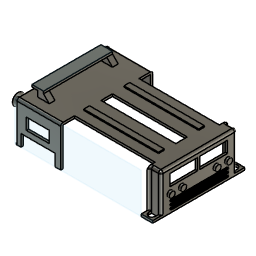
coverrrrr v1 v2 (Autodesk Fusion 360 design; units mm, degrees)
Autodesk Fusion 360 part; units mm, degrees
note: some values were not read from the file. Set by a fixed rule: which sketch regions a step uses.
sketch "Sketch1" plane through (0, 0, 0) normal (0, 0, 1) x (1, 0, 0)
  line L0 (0, 0) -> (120, 0)
  line L1 (120, 0) -> (120, 80)
  line L2 (120, 80) -> (0, 80)
  line L3 (0, 80) -> (0, 0)
  dimension "d1" = 120
  dimension "d2" = 80
  constraint horizontal L0
  constraint vertical L1
  constraint horizontal L2
  constraint vertical L3
  constraint coincident L0.start L3.end
  measures "d1" distance of L0.start L0.end
  measures "d2" distance of L0.start L2.end
extrude "Extrude1" add sketch "Sketch1" along normal blind 35
sketch "Sketch2" plane through (0, 0, 35) normal (0, 0, 1) x (-1, 0, 0)
  line L0 (0, -80) -> (0, 0)
  line L1 (0, 0) -> (-120, 0)
  line L2 (-120, 0) -> (-120, -80)
  line L3 (-120, -80) -> (0, -80)
  line L4 (-120, 0) -> (-110, 0)
  line L5 (-110, 0) -> (-110, -7)
  line L6 (-110, -7) -> (-120, -7)
  line L7 (-120, -7) -> (-120, 0)
  dimension "d5" = 10
  dimension "d6" = 7
  constraint horizontal L4
  constraint vertical L5
  constraint horizontal L6
  constraint vertical L7
  constraint coincident L1.end L2.start
  measures "d5" distance of L1.end L4.end
  measures "d6" distance of L1.end L6.end
extrude "Extrude2" cut sketch "Sketch2" against normal blind 33 contours L1 L2 L4 L5 L6 L7
sketch "Sketch3" plane through (0, 0, 35) normal (0, 0, 1) x (-1, 0, 0)
  line L0 (-110, 0) -> (-110, -7)
  line L1 (-110, -7) -> (-120, -7)
  line L2 (-120, -7) -> (-120, -80)
  line L3 (-120, -80) -> (0, -80)
  line L4 (0, -80) -> (0, 0)
  line L5 (0, 0) -> (-110, 0)
  line L6 (-120, -80) -> (-110, -80)
  line L7 (-110, -80) -> (-110, -73)
  line L8 (-110, -73) -> (-120, -73)
  line L9 (-120, -73) -> (-120, -80)
  dimension "d9" = 10
  dimension "d10" = 7
  constraint horizontal L6
  constraint vertical L7
  constraint horizontal L8
  constraint vertical L9
  constraint coincident L2.end L3.start
  measures "d9" distance of L2.end L6.end
  measures "d10" distance of L2.end L8.end
extrude "Extrude3" cut sketch "Sketch3" against normal blind 33 contours L2 L3 L6 L7 L8 L9
sketch "Sketch4" plane through (0, 0, 2) normal (0, 0, 1) x (-1, 0, 0)
  line L0 (-120, -7) -> (-110, -7)
  line L1 (-110, -7) -> (-110, 0)
  line L2 (-110, 0) -> (-120, 0)
  line L3 (-120, 0) -> (-120, -7)
  line L4 (-110, -2) -> (-113, -2)
  line L5 (-113, -2) -> (-113, 0)
  circle A0 centre (-115, -4) radius 2.75
  dimension "d13" = 5.5
  constraint coincident L1 L4.start
  constraint perpendicular L1 L4
  constraint coincident L2 L5.end
  constraint perpendicular L2 L5
  measures "d13" diameter of A0
extrude "Extrude4" cut sketch "Sketch4" against normal blind 5 contours A0
sketch "Sketch5" plane through (0, 0, 2) normal (0, 0, 1) x (-1, 0, 0)
  line L0 (-120, -73) -> (-120, -80)
  line L1 (-120, -80) -> (-110, -80)
  line L2 (-110, -80) -> (-110, -73)
  line L3 (-110, -73) -> (-120, -73)
  line L4 (-110, -78) -> (-113, -78)
  line L5 (-113, -78) -> (-113, -80)
  circle A0 centre (-115, -76) radius 2.75
  dimension "d16" = 5.5
  constraint coincident L2 L4.start
  constraint perpendicular L2 L4
  constraint coincident L1 L5.end
  constraint perpendicular L1 L5
  measures "d16" diameter of A0
extrude "Extrude5" cut sketch "Sketch5" against normal blind 4 contours A0
sketch "Sketch6" plane through (0, 0, 0) normal (0, -1, 0) x (1, 0, 0)
  line L0 (110, 2) -> (110, 35)
  line L1 (110, 35) -> (0, 35)
  line L2 (0, 35) -> (0, 0)
  line L3 (0, 0) -> (120, 0)
  line L4 (120, 0) -> (120, 2)
  line L5 (120, 2) -> (110, 2)
shell "Shell1" thickness 2 removed faces 1 at (37.5759, 28.5164, 0)
sketch "Sketch7" plane through (0, 0, 0) normal (0, -1, 0) x (1, 0, 0)
sketch "Sketch8" plane through (0, 0, 0) normal (0, -1, 0) x (1, 0, 0)
  line L0 (0, 0) -> (40, 0)
  line L1 (40, 0) -> (105, 0)
  line L2 (105, 0) -> (105, 25)
  line L3 (105, 25) -> (40, 25)
  line L4 (40, 25) -> (40, 0)
  dimension "d20" = 40
  dimension "d21" = 65
  dimension "d22" = 25
  constraint coincident L0.start origin
  constraint horizontal L0
  constraint horizontal L1
  constraint vertical L2
  constraint horizontal L3
  constraint vertical L4
  measures "d20" distance of L0.start L0.end
  measures "d21" distance of L0.end L1.end
  measures "d22" distance of L0.end L3.end
extrude "Extrude6" cut sketch "Sketch8" against normal blind 150
sketch "Sketch9" plane through (0, 0, 0) normal (-1, 0, 0) x (0, -1, 0)
  line L0 (-80, 0) -> (0, 0)
  line L1 (0, 0) -> (0, 35)
  line L2 (0, 35) -> (-80, 35)
  line L3 (-80, 35) -> (-80, 0)
  line L4 (-5, 0) -> (-75, 0)
  line L5 (-75, 0) -> (-75, 30)
  line L6 (-75, 30) -> (-5, 30)
  line L7 (-5, 30) -> (-5, 0)
  constraint horizontal L4
  constraint vertical L5
  constraint horizontal L6
  constraint vertical L7
  constraint coincident L0 L4.start
extrude "Extrude7" cut sketch "Sketch9" against normal blind 15 contours L0 L4 L5 L6 L7
fillet "Fillet1" radius 10 6 edges at (105, 1, 25) (40, 1, 25) (40, 79, 25) (105, 79, 25) (1, 5, 30) (1, 75, 30)
fillet "Fillet2" radius 2 16 edges at (55, 80, 35) (0, 80, 17.5) (0, 40, 35) (0, 0, 17.5) (55, 0, 35) (110, 3.5, 35) (115, 7, 35) (120, 40, 35) (115, 73, 35) (110, 76.5, 35) (120, 73, 18.5) (110, 80, 18.5) (110, 73, 18.5) (110, 0, 18.5) (110, 7, 18.5) (120, 7, 18.5)
sketch "Sketch10" plane through (0, 0, 35) normal (0, 0, 1) x (-1, 0, 0)
  arc A0 (-108, -75) -> (-112, -71) centre (-112, -75) ccw
  line L0 (-108, -75) -> (-108, -78)
  line L1 (-108, -78) -> (-2, -78)
  line L2 (-2, -78) -> (-2, -2)
  line L3 (-2, -2) -> (-108, -2)
  line L4 (-108, -2) -> (-108, -5)
  arc A1 (-112, -9) -> (-108, -5) centre (-112, -5) ccw
  line L5 (-112, -9) -> (-118, -9)
  line L6 (-118, -9) -> (-118, -71)
  line L7 (-118, -71) -> (-112, -71)
  line L8 (-20, -10) -> (-10, -10)
  line L9 (-10, -10) -> (-10, -15)
  line L10 (-10, -15) -> (-20, -15)
  line L11 (-20, -15) -> (-20, -10)
  line L12 (-20, -65) -> (-10, -65)
  line L13 (-10, -65) -> (-10, -70)
  line L14 (-10, -70) -> (-20, -70)
  line L15 (-20, -70) -> (-20, -65)
  constraint horizontal L8
  constraint vertical L9
  constraint horizontal L10
  constraint vertical L11
  constraint horizontal L12
  constraint vertical L13
  constraint horizontal L14
  constraint vertical L15
extrude "Extrude8" add sketch "Sketch10" along normal blind 5 contours L8 L9 L10 L11 | L12 L13 L14 L15
sketch "Sketch11" plane through (0, 0, 40) normal (0, 0, 1) x (-1, 0, 0)
  line L0 (-20, -15) -> (-10, -15)
  line L1 (-10, -15) -> (-10, -10)
  line L2 (-10, -10) -> (-20, -10)
  line L3 (-20, -10) -> (-20, -15)
  line L4 (-15, -10) -> (-5, -10)
  line L5 (-5, -10) -> (-5, -70)
  line L6 (-5, -70) -> (-15, -70)
  line L7 (-15, -70) -> (-15, -10)
  constraint horizontal L4
  constraint vertical L5
  constraint horizontal L6
  constraint vertical L7
  constraint midpoint L2 L4.start
extrude "Extrude9" add sketch "Sketch11" along normal blind 2 contours L0 L1 L2 L4 L7 | L0 L1 L4 L5 L6 L7
sketch "Sketch12" plane through (0, 0, 0) normal (0, -1, 0) x (1, 0, 0)
  line L0 (40, 30) -> (100, 30)
  line L1 (100, 30) -> (100, 28)
  line L2 (100, 28) -> (40, 28)
  line L3 (40, 28) -> (40, 30)
  constraint horizontal L0
  constraint vertical L1
  constraint horizontal L2
  constraint vertical L3
sketch "Sketch13" plane through (0, 80, 0) normal (0, 1, 0) x (-1, 0, 0)
  line L0 (-2, 0) -> (-2, 33)
  line L1 (-2, 33) -> (-108, 33)
  line L2 (-108, 33) -> (-108, 2)
  line L3 (-108, 2) -> (-120, 2)
  line L4 (-120, 2) -> (-120, 0)
  line L5 (-120, 0) -> (-105, 0)
  line L6 (-105, 0) -> (-105, 15)
  arc A0 (-95, 25) -> (-105, 15) centre (-95, 15) ccw
  line L7 (-95, 25) -> (-50, 25)
  arc A1 (-40, 15) -> (-50, 25) centre (-50, 15) ccw
  line L8 (-40, 15) -> (-40, 0)
  line L9 (-40, 0) -> (-2, 0)
  line L10 (-40, 30) -> (-100, 30)
  line L11 (-100, 30) -> (-100, 28)
  line L12 (-100, 28) -> (-40, 28)
  line L13 (-40, 28) -> (-40, 30)
  constraint horizontal L10
  constraint vertical L11
  constraint horizontal L12
  constraint vertical L13
extrude "Extrude10" add sketch "Sketch12" along normal blind 20
extrude "Extrude11" add sketch "Sketch13" along normal blind 20 contours L10 L11 L12 L13
sketch "Sketch14" plane through (0, 0, 30) normal (0, 0, 1) x (-1, 0, 0)
  line L0 (-40, -80) -> (-100, -80)
  line L1 (-100, -80) -> (-100, -100)
  line L2 (-100, -100) -> (-40, -100)
  line L3 (-40, -100) -> (-40, -80)
  line L4 (-100, 0) -> (-40, 20)
  line L5 (-40, 20) -> (-100, 20)
  line L6 (-100, 20) -> (-100, 0)
  line L7 (-100, -80) -> (-40, -100)
  line L8 (-100, -100) -> (-100, -80)
  constraint horizontal L5
  constraint perpendicular L5 L6
  constraint coincident L0.end L1.start
  constraint coincident L2.end L3.start
  constraint coincident L1.end L2.start
extrude "Extrude12" cut sketch "Sketch14" against normal blind 10 contours L1 L2 L7 L8 | L4 L5 L6
sketch "Sketch15" plane through (0, 0, 30) normal (0, 0, 1) x (-1, 0, 0)
  line L0 (-100, -80) -> (-40, -100)
  line L1 (-40, -100) -> (-40, -80)
  line L2 (-40, -80) -> (-100, -80)
  circle A0 centre (-40, -90) radius 10
  circle A1 centre (-40, 10) radius 10
  constraint midpoint L1 A0.centre
  constraint coincident L1.end A0
extrude "Extrude13" cut sketch "Sketch15" against normal blind 10 contours L0 L1 A0 | L1 A0 | A1
sketch "Sketch16" plane through (0, 0, 0) normal (-1, 0, 0) x (0, -1, 0)
  line L0 (-78, 33) -> (-78, 0)
  line L1 (-78, 0) -> (-75, 0)
  line L2 (-75, 0) -> (-75, 20)
  arc A0 (-65, 30) -> (-75, 20) centre (-65, 20) ccw
  line L3 (-65, 30) -> (-15, 30)
  arc A1 (-5, 20) -> (-15, 30) centre (-15, 20) ccw
  line L4 (-5, 20) -> (-5, 0)
  line L5 (-5, 0) -> (-2, 0)
  line L6 (-2, 0) -> (-2, 33)
  line L7 (-2, 33) -> (-78, 33)
  circle A2 centre (-72.0711, 27.0711) radius 5
  circle A3 centre (-7.9289, 27.0711) radius 5
  dimension "d43" = 10
  dimension "d44" = 10
  constraint midpoint A0 A2.centre
  constraint midpoint A1 A3.centre
  measures "d43" diameter of A2
  measures "d44" diameter of A3
extrude "Extrude14" add sketch "Sketch16" along normal blind 5 contours A0 A2 | A0 A2 | A1 A3 | A1 A3
sketch "Sketch17" plane through (120, 0, 0) normal (1, 0, 0) x (0, 1, 0)
  line L0 (80, 2) -> (71, 2)
  line L1 (71, 2) -> (71, 33)
  line L2 (71, 33) -> (9, 33)
  line L3 (9, 33) -> (9, 2)
  line L4 (9, 2) -> (0, 2)
  line L5 (0, 2) -> (0, 0)
  line L6 (0, 0) -> (80, 0)
  line L7 (80, 0) -> (80, 2)
  line L8 (15, 30) -> (65, 30)
  line L9 (65, 30) -> (65, 20)
  line L10 (65, 20) -> (15, 20)
  line L11 (15, 20) -> (15, 30)
  constraint horizontal L8
  constraint vertical L9
  constraint horizontal L10
  constraint vertical L11
extrude "Extrude15" cut sketch "Sketch17" against normal blind 10 contours L8 L9 L10 L11
sketch "Sketch18" plane through (120, 0, 0) normal (1, 0, 0) x (0, 1, 0)
  line L0 (65, 30) -> (65, 20)
  line L1 (65, 20) -> (15, 20)
  line L2 (15, 20) -> (15, 30)
  line L3 (15, 30) -> (65, 30)
  line L4 (80, 2) -> (71, 2)
  line L5 (71, 2) -> (71, 33)
  line L6 (71, 33) -> (9, 33)
  line L7 (9, 33) -> (9, 2)
  line L8 (9, 2) -> (0, 2)
  line L9 (0, 2) -> (0, 0)
  line L10 (0, 0) -> (80, 0)
  line L11 (80, 0) -> (80, 2)
  circle A0 centre (15, 15) radius 2.5
  circle A1 centre (25, 15) radius 2.5
  circle A2 centre (65, 15) radius 2.5
  circle A3 centre (55, 15) radius 2.5
  dimension "d49" = 5
  dimension "d50" = 5
  dimension "d51" = 5
  dimension "d52" = 5
  measures "d49" diameter of A0
  measures "d50" diameter of A1
  measures "d51" diameter of A2
  measures "d52" diameter of A3
extrude "Extrude16" add sketch "Sketch18" along normal blind 2 contours A0 | A1 | A2 | A3
sketch "Sketch19" plane through (120, 0, 0) normal (1, 0, 0) x (0, 1, 0)
  circle A0 centre (65, 15) radius 2.5
  circle A1 centre (15, 15) radius 2.5
  circle A2 centre (55, 15) radius 2.5
  circle A3 centre (25, 15) radius 2.5
  line L0 (65, 30) -> (65, 20)
  line L1 (65, 20) -> (15, 20)
  line L2 (15, 20) -> (15, 30)
  line L3 (15, 30) -> (65, 30)
  line L4 (80, 2) -> (71, 2)
  line L5 (71, 2) -> (71, 33)
  line L6 (71, 33) -> (9, 33)
  line L7 (9, 33) -> (9, 2)
  line L8 (9, 2) -> (0, 2)
  line L9 (0, 2) -> (0, 0)
  line L10 (0, 0) -> (80, 0)
  line L11 (80, 0) -> (80, 2)
sketch "Sketch20" plane through (120, 0, 0) normal (1, 0, 0) x (0, 1, 0)
  line L0 (15, 10) -> (65, 10)
  line L1 (65, 10) -> (65, 9)
  line L2 (65, 9) -> (15, 9)
  line L3 (15, 9) -> (15, 10)
  line L4 (65, 7) -> (15, 7)
  line L5 (15, 7) -> (15, 6)
  line L6 (15, 6) -> (65, 6)
  line L7 (65, 6) -> (65, 7)
  line L8 (15, 4) -> (65, 4)
  line L9 (65, 4) -> (65, 3)
  line L10 (65, 3) -> (15, 3)
  line L11 (15, 3) -> (15, 4)
  constraint horizontal L0
  constraint vertical L1
  constraint horizontal L2
  constraint vertical L3
  constraint horizontal L4
  constraint vertical L5
  constraint horizontal L6
  constraint vertical L7
  constraint horizontal L8
  constraint vertical L9
  constraint horizontal L10
  constraint vertical L11
extrude "Extrude17" add sketch "Sketch20" along normal blind 1
sketch "Sketch21" plane through (0, 0, 20) normal (0, 0, 1) x (-1, 0, 0)
  line L0 (-118, -65) -> (-118, -15)
  line L1 (-118, -15) -> (-120, -15)
  line L2 (-120, -15) -> (-120, -65)
  line L3 (-120, -65) -> (-118, -65)
  line L4 (-118, -27) -> (-118, -53)
  line L5 (-120, -27) -> (-120, -40)
  line L6 (-118, -39) -> (-120, -39)
  line L7 (-120, -39) -> (-120, -41)
  line L8 (-120, -41) -> (-118, -41)
  line L9 (-118, -41) -> (-118, -39)
  constraint coincident L0 L4.start
  constraint coincident L0 L4.end
  constraint coincident L2 L5.start
  constraint midpoint L2 L5.end
  constraint horizontal L6
  constraint vertical L7
  constraint horizontal L8
  constraint vertical L9
  constraint coincident L2 L7.end
  constraint coincident L4 L6.start
extrude "Extrude18" add sketch "Sketch21" along normal blind 10 contours L0 L2 L4 L5 L6 L7 L8 L9
sketch "Sketch22" plane through (0, 0, 35) normal (0, 0, 1) x (-1, 0, 0)
  line L0 (-20, -15) -> (-20, -10)
  line L1 (-20, -10) -> (-10, -10)
  line L2 (-10, -10) -> (-10, -15)
  line L3 (-10, -15) -> (-20, -15)
  line L4 (-20, -70) -> (-20, -65)
  line L5 (-20, -65) -> (-10, -65)
  line L6 (-10, -65) -> (-10, -70)
  line L7 (-10, -70) -> (-20, -70)
  arc A0 (-108, -75) -> (-112, -71) centre (-112, -75) ccw
  line L8 (-108, -75) -> (-108, -78)
  line L9 (-108, -78) -> (-2, -78)
  line L10 (-2, -78) -> (-2, -2)
  line L11 (-2, -2) -> (-108, -2)
  line L12 (-108, -2) -> (-108, -5)
  arc A1 (-112, -9) -> (-108, -5) centre (-112, -5) ccw
  line L13 (-112, -9) -> (-118, -9)
  line L14 (-118, -9) -> (-118, -71)
  line L15 (-118, -71) -> (-112, -71)
  line L16 (-40, -60) -> (-105, -60)
  line L17 (-105, -60) -> (-105, -55)
  line L18 (-105, -55) -> (-40, -55)
  line L19 (-40, -55) -> (-40, -60)
  line L20 (-40, -20) -> (-105, -20)
  line L21 (-105, -20) -> (-105, -25)
  line L22 (-105, -25) -> (-40, -25)
  line L23 (-40, -25) -> (-40, -20)
  constraint horizontal L16
  constraint vertical L17
  constraint horizontal L18
  constraint vertical L19
  constraint horizontal L20
  constraint vertical L21
  constraint horizontal L22
  constraint vertical L23
extrude "Extrude19" add sketch "Sketch22" along normal blind 1 contours L16 L17 L18 L19 | L20 L21 L22 L23
sketch "Sketch23" plane through (-5, 0, 0) normal (-1, 0, 0) x (0, -1, 0)
  circle A0 centre (-7.9289, 27.0711) radius 5
  circle A1 centre (-7.9289, 27.0711) radius 4
  dimension "d61" = 8
  constraint concentric A0 A1
  measures "d61" diameter of A1
extrude "Extrude20" cut sketch "Sketch23" against normal blind 4 contours A1
sketch "Sketch24" plane through (-5, 0, 0) normal (-1, 0, 0) x (0, -1, 0)
  circle A0 centre (-72.0711, 27.0711) radius 5
  circle A1 centre (-72.0711, 27.0711) radius 4
  dimension "d64" = 8
  constraint concentric A0 A1
  measures "d64" diameter of A1
extrude "Extrude21" cut sketch "Sketch24" against normal blind 4 contours A1
sketch "Sketch25" plane through (0, 10, 0) normal (0, -1, 0) x (1, 0, 0)
  line L0 (10, 35) -> (20, 35)
  line L1 (20, 35) -> (20, 40)
  line L2 (20, 40) -> (15, 40)
  line L3 (15, 40) -> (15, 42)
  line L4 (15, 42) -> (5, 42)
  line L5 (5, 42) -> (5, 40)
  line L6 (5, 40) -> (10, 40)
  line L7 (10, 40) -> (10, 35)
  line L8 (15, 40) -> (20, 35)
  line L9 (20, 40) -> (15, 40)
  constraint coincident L2.end L3.start
  constraint coincident L0.end L1.start
  constraint coincident L1.end L2.start
extrude "Extrude22" cut sketch "Sketch25" against normal blind 63 contours L1 L2 L8 L9
sketch "Sketch26" plane through (0, 0, 42) normal (0, 0, 1) x (-1, 0, 0)
  line L0 (-15, -70) -> (-5, -70)
  line L1 (-5, -70) -> (-5, -10)
  line L2 (-5, -10) -> (-15, -10)
  line L3 (-15, -10) -> (-15, -70)
extrude "Extrude23" cut 2 faces at (66.5474, -5.5104, 30) (66.5474, 85.5104, 30) along direction (0, 0, -1) blind 10
sketch "Sketch27" plane through (0, 80, 0) normal (0, 1, 0) x (-1, 0, 0)
  arc A0 (-40, 15) -> (-50, 25) centre (-50, 15) ccw
  line L0 (-40, 15) -> (-40, 0)
  line L1 (-40, 0) -> (-2, 0)
  line L2 (-2, 0) -> (-2, 33)
  line L3 (-2, 33) -> (-108, 33)
  line L4 (-108, 33) -> (-108, 2)
  line L5 (-108, 2) -> (-120, 2)
  line L6 (-120, 2) -> (-120, 0)
  line L7 (-120, 0) -> (-105, 0)
  line L8 (-105, 0) -> (-105, 15)
  arc A1 (-95, 25) -> (-105, 15) centre (-95, 15) ccw
  line L9 (-95, 25) -> (-50, 25)
  line L10 (-30, 25) -> (-10, 25)
  line L11 (-10, 25) -> (-10, 15)
  line L12 (-10, 15) -> (-30, 15)
  line L13 (-30, 15) -> (-30, 25)
  constraint horizontal L10
  constraint vertical L11
  constraint horizontal L12
  constraint vertical L13
extrude "Extrude24" cut sketch "Sketch27" against normal blind 90 contours L10 L11 L12 L13
sketch "Sketch28" plane through (0, 0, 35) normal (0, 0, 1) x (-1, 0, 0)
  line L0 (-20, -65) -> (-10, -65)
  line L1 (-10, -65) -> (-10, -70)
  line L2 (-10, -70) -> (-20, -70)
  line L3 (-20, -70) -> (-20, -65)
  line L4 (-40, -55) -> (-40, -60)
  line L5 (-40, -60) -> (-105, -60)
  line L6 (-105, -60) -> (-105, -55)
  line L7 (-105, -55) -> (-40, -55)
  line L8 (-40, -25) -> (-105, -25)
  line L9 (-105, -25) -> (-105, -20)
  line L10 (-105, -20) -> (-40, -20)
  line L11 (-40, -20) -> (-40, -25)
  line L12 (-20, -15) -> (-20, -10)
  line L13 (-20, -10) -> (-10, -10)
  line L14 (-10, -10) -> (-10, -15)
  line L15 (-10, -15) -> (-20, -15)
  arc A0 (-108, -75) -> (-112, -71) centre (-112, -75) ccw
  line L16 (-108, -75) -> (-108, -78)
  line L17 (-108, -78) -> (-2, -78)
  line L18 (-2, -78) -> (-2, -2)
  line L19 (-2, -2) -> (-108, -2)
  line L20 (-108, -2) -> (-108, -5)
  arc A1 (-112, -9) -> (-108, -5) centre (-112, -5) ccw
  line L21 (-112, -9) -> (-118, -9)
  line L22 (-118, -9) -> (-118, -71)
  line L23 (-118, -71) -> (-112, -71)
  line L24 (-40, -45) -> (-105, -45)
  line L25 (-105, -45) -> (-105, -35)
  line L26 (-105, -35) -> (-40, -35)
  line L27 (-40, -35) -> (-40, -45)
  constraint horizontal L24
  constraint vertical L25
  constraint horizontal L26
  constraint vertical L27
extrude "Extrude25" cut sketch "Sketch28" against normal blind 5 contours L24 L25 L26 L27
sketch "Sketch29" plane through (0, 0, 0) normal (0, -1, 0) x (1, 0, 0)
  line L0 (40, 0) -> (110, 0)
  line L1 (110, 0) -> (110, 40)
  line L2 (110, 40) -> (40, 40)
  line L3 (40, 40) -> (40, 0)
  constraint horizontal L0
  constraint vertical L1
  constraint horizontal L2
  constraint vertical L3
extrude "Extrude26" cut sketch "Sketch29" against normal blind 12
sketch "Sketch30" plane through (0, 80, 0) normal (0, 1, 0) x (-1, 0, 0)
  line L0 (-10, 25) -> (-10, 15)
  line L1 (-10, 15) -> (-30, 15)
  line L2 (-30, 15) -> (-30, 25)
  line L3 (-30, 25) -> (-10, 25)
  arc A0 (-40, 15) -> (-50, 25) centre (-50, 15) ccw
  line L4 (-40, 15) -> (-40, 0)
  line L5 (-40, 0) -> (-2, 0)
  line L6 (-2, 0) -> (-2, 33)
  line L7 (-2, 33) -> (-108, 33)
  line L8 (-108, 33) -> (-108, 2)
  line L9 (-108, 2) -> (-120, 2)
  line L10 (-120, 2) -> (-120, 0)
  line L11 (-120, 0) -> (-105, 0)
  line L12 (-105, 0) -> (-105, 15)
  arc A1 (-95, 25) -> (-105, 15) centre (-95, 15) ccw
  line L13 (-95, 25) -> (-50, 25)
  line L14 (-40, 0) -> (-110, 0)
  line L15 (-110, 0) -> (-110, 40)
  line L16 (-110, 40) -> (-40, 40)
  line L17 (-40, 40) -> (-40, 0)
  constraint horizontal L14
  constraint vertical L15
  constraint horizontal L16
  constraint vertical L17
  constraint coincident L4.end L5.start
extrude "Extrude27" cut sketch "Sketch30" against normal blind 12 contours A0 L4 L12 A1 L13 L14 L17 | A0 L7 L8 L9 L11 L12 A1 L13 L14 L15 L17 | L7 L8 L9 L15 L16 L17
sketch "Sketch31" plane through (0, 80, 0) normal (0, 1, 0) x (-1, 0, 0)
  line L0 (-10, 25) -> (-10, 15)
  line L1 (-10, 15) -> (-30, 15)
  line L2 (-30, 15) -> (-30, 25)
  line L3 (-30, 25) -> (-10, 25)
  line L4 (-40, 33) -> (-40, 0)
  line L5 (-40, 0) -> (-2, 0)
  line L6 (-2, 0) -> (-2, 33)
  line L7 (-2, 33) -> (-40, 33)
  line L8 (-35.0239, 0) -> (-5.4624, 0)
  line L9 (-5.4624, 0) -> (-5.4624, 10.2822)
  line L10 (-5.4624, 10.2822) -> (-35.0239, 10.2822)
  line L11 (-35.0239, 10.2822) -> (-35.0239, 0)
  constraint horizontal L8
  constraint vertical L9
  constraint horizontal L10
  constraint vertical L11
  constraint coincident L5 L8.start
extrude "Extrude28" cut sketch "Sketch31" against normal blind 150 contours L5 L8 L9 L10 L11
sketch "Sketch32" plane through (0, 0, 2) normal (0, 0, 1) x (-1, 0, 0)
  line L0 (-110, -80) -> (-110, -75)
  arc A0 (-110, -75) -> (-112, -73) centre (-112, -75) ccw
  line L1 (-112, -73) -> (-118, -73)
  arc A1 (-120, -71) -> (-118, -73) centre (-118, -71) ccw
  line L2 (-120, -71) -> (-120, -80)
  line L3 (-120, -80) -> (-110, -80)
  circle A2 centre (-115, -76) radius 2.75
  line L4 (-118, -73) -> (-112, -73)
  line L5 (-112, -73) -> (-112, -76)
  line L6 (-112, -76) -> (-118, -76)
  line L7 (-118, -76) -> (-118, -73)
  line L8 (-118, -7) -> (-112, -7)
  line L9 (-112, -7) -> (-112, -4)
  line L10 (-112, -4) -> (-118, -4)
  line L11 (-118, -4) -> (-118, -7)
  constraint horizontal L4
  constraint vertical L5
  constraint horizontal L6
  constraint vertical L7
  constraint coincident L1.end A1.end
  constraint horizontal L8
  constraint vertical L9
  constraint horizontal L10
  constraint vertical L11
extrude "Extrude29" cut sketch "Sketch32" against normal blind 4 contours L1 A2 L4 L5 L6 L7 | A2 L6 | L8 L9 L10 L11 picked at (-114.9315, -75.0859)
